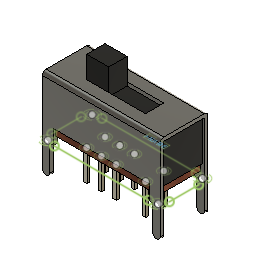
Switch-EG2301 v5 (Autodesk Fusion 360 design; units mm, degrees)
Autodesk Fusion 360 part; units mm, degrees
sketch "Sketch1" plane through (0, 0, 0) normal (0, 0, 1) x (1, 0, 0)
  line L0 (-4.25, 1.45) -> (-3.75, 1.45)
  line L1 (-3.75, 1.45) -> (-3.75, 1.05)
  line L2 (-3.75, 1.05) -> (-4.25, 1.05)
  line L3 (-4.25, 1.05) -> (-4.25, 1.45)
  line L4 (-2.25, 1.45) -> (-1.75, 1.45)
  line L5 (-1.75, 1.45) -> (-1.75, 1.05)
  line L6 (-1.75, 1.05) -> (-2.25, 1.05)
  line L7 (-2.25, 1.05) -> (-2.25, 1.45)
  line L8 (-0.25, 1.45) -> (0.25, 1.45)
  line L9 (0.25, 1.45) -> (0.25, 1.05)
  line L10 (0.25, 1.05) -> (-0.25, 1.05)
  line L11 (-0.25, 1.05) -> (-0.25, 1.45)
  line L12 (3.75, 1.45) -> (4.25, 1.45)
  line L13 (4.25, 1.45) -> (4.25, 1.05)
  line L14 (4.25, 1.05) -> (3.75, 1.05)
  line L15 (3.75, 1.05) -> (3.75, 1.45)
  line L16 (-8, 3.25) -> (-7, 3.25)
  line L17 (-7, 3.25) -> (-7, 2.75)
  line L18 (-7, 2.75) -> (-8, 2.75)
  line L19 (-8, 2.75) -> (-8, 3.25)
  line L20 (7, 3.25) -> (8, 3.25)
  line L21 (8, 3.25) -> (8, 2.75)
  line L22 (8, 2.75) -> (7, 2.75)
  line L23 (7, 2.75) -> (7, 3.25)
  line L24 (0, 0) -> (8, 0) construction
  line L25 (0.25, -1.45) -> (0.25, -1.05)
  line L26 (-2.25, -1.45) -> (-1.75, -1.45)
  line L27 (-0.25, -1.05) -> (-0.25, -1.45)
  line L28 (-8, -3.25) -> (-7, -3.25)
  line L29 (-3.75, -1.05) -> (-4.25, -1.05)
  line L30 (7, -3.25) -> (8, -3.25)
  line L31 (8, -2.75) -> (7, -2.75)
  line L32 (7, -2.75) -> (7, -3.25)
  line L33 (3.75, -1.05) -> (3.75, -1.45)
  line L34 (8, -3.25) -> (8, -2.75)
  line L35 (-0.25, -1.45) -> (0.25, -1.45)
  line L36 (-7, -2.75) -> (-8, -2.75)
  line L37 (-2.25, -1.05) -> (-2.25, -1.45)
  line L38 (-3.75, -1.45) -> (-3.75, -1.05)
  line L39 (-4.25, -1.45) -> (-3.75, -1.45)
  line L40 (-4.25, -1.05) -> (-4.25, -1.45)
  line L41 (0.25, -1.05) -> (-0.25, -1.05)
  line L42 (-7, -3.25) -> (-7, -2.75)
  line L43 (-1.75, -1.05) -> (-2.25, -1.05)
  line L44 (3.75, -1.45) -> (4.25, -1.45)
  line L45 (-8, -2.75) -> (-8, -3.25)
  line L46 (4.25, -1.05) -> (3.75, -1.05)
  line L47 (-1.75, -1.45) -> (-1.75, -1.05)
  line L48 (4.25, -1.45) -> (4.25, -1.05)
  dimension "d1" = 0.5
  dimension "d2" = 1
  dimension "d3" = 1
  dimension "d4" = 0.5
  dimension "d5" = 0.5
  dimension "d6" = 0.4
  dimension "d7" = 0.5
  dimension "d8" = 0.4
  dimension "d9" = 0.5
  dimension "d10" = 0.4
  dimension "d11" = 0.5
  dimension "d12" = 0.4
  dimension "d13" = 0.25
  dimension "d14" = 1.05
  dimension "d15" = 4.25
  dimension "d16" = 1.75
  dimension "d17" = 3.75
  dimension "d18" = 7
  dimension "d19" = 8
  dimension "d20" = 2.75
  constraint horizontal L0
  constraint vertical L1
  constraint horizontal L2
  constraint vertical L3
  constraint horizontal L4
  constraint vertical L5
  constraint horizontal L6
  constraint vertical L7
  constraint horizontal L8
  constraint vertical L9
  constraint horizontal L10
  constraint vertical L11
  constraint horizontal L12
  constraint vertical L13
  constraint horizontal L14
  constraint vertical L15
  constraint horizontal L16
  constraint vertical L17
  constraint horizontal L18
  constraint vertical L19
  constraint horizontal L20
  constraint vertical L21
  constraint horizontal L22
  constraint vertical L23
  constraint collinear L0 L4
  constraint collinear L4 L8
  constraint collinear L8 L12
  constraint collinear L16 L20
  constraint coincident L24.start origin
  constraint perpendicular L11 L24
  constraint symmetric L0.start L24 L39.start
  constraint symmetric L0.end L24 L38.start
  constraint symmetric L1.end L24 L29.start
  constraint symmetric L2.end L24 L29.end
  constraint symmetric L4.start L24 L26.start
  constraint symmetric L4.end L24 L26.end
  constraint symmetric L5.end L24 L43.start
  constraint symmetric L6.end L24 L37.start
  constraint symmetric L8.start L24 L27.end
  constraint symmetric L8.end L24 L25.start
  constraint symmetric L9.end L24 L25.end
  constraint symmetric L10.end L24 L27.start
  constraint symmetric L12.start L24 L33.end
  constraint symmetric L12.end L24 L44.end
  constraint symmetric L13.end L24 L46.start
  constraint symmetric L14.end L24 L33.start
  constraint symmetric L16.start L24 L28.start
  constraint symmetric L16.end L24 L28.end
  constraint symmetric L17.end L24 L36.start
  constraint symmetric L18.end L24 L36.end
  constraint symmetric L20.start L24 L30.start
  constraint symmetric L20.end L24 L30.end
  constraint symmetric L21.end L24 L31.start
  constraint symmetric L22.end L24 L31.end
  measures "d1" distance of L16.end L17.end
  measures "d2" distance of L16.start L16.end
  measures "d3" distance of L20.start L20.end
  measures "d4" distance of L20.end L21.end
  measures "d5" distance of L12.start L12.end
  measures "d6" distance of L12.end L13.end
  measures "d7" distance of L8.start L8.end
  measures "d8" distance of L8.end L9.end
  measures "d9" distance of L4.start L4.end
  measures "d10" distance of L4.end L5.end
  measures "d11" distance of L0.start L0.end
  measures "d12" distance of L0.end L1.end
  measures "d13" distance of L24.start L9
  measures "d14" distance of L24.start L10
  measures "d15" distance of L24.start L13
  measures "d16" distance of L24.start L5
  measures "d17" distance of L24.start L1
  measures "d18" distance of L24.start L17
  measures "d19" distance of L24.start L21
  measures "d20" distance of L24.start L22
extrude "Extrude1" add sketch "Sketch1" against normal blind 4 makes body 1 at (-0.0833, -1.45, -1.3333) makes body 2 at (7.6667, 2.75, -1.3333) makes body 3 at (-4.0833, 1.45, -1.3333) makes body 4 at (-2.0833, 1.45, -1.3333) makes body 5 at (-7.6667, -3.25, -1.3333) makes body 6 at (4.0833, -1.05, -1.3333) makes body 7 at (-2.0833, -1.45, -1.3333) makes body 8 at (4.0833, 1.05, -1.3333) makes body 9 at (-7.6667, 3.25, -1.3333) makes body 10 at (-0.0833, 1.45, -1.3333) makes body 11 at (-4.0833, -1.45, -1.3333) makes body 12 at (7.6667, -2.75, -1.3333)
fillet "Fillet1" radius 0.5 8 edges at (8, 3, -4) (7, 3, -4) (-7, -3, -4) (-8, -3, -4) (-7, 3, -4) (-8, 3, -4) (8, -3, -4) (7, -3, -4) on bodies 2 5 9 12
sketch "Sketch2" plane through (0, 0, 0) normal (0, 0, 1) x (1, 0, 0)
  line L0 (-8, 2.75) -> (-7, 2.75)
  line L1 (-7, 2.75) -> (-7, 3.25)
  line L2 (-7, 3.25) -> (-8, 3.25)
  line L3 (-8, 3.25) -> (-8, 2.75)
  line L4 (-4.25, 1.05) -> (-3.75, 1.05)
  line L5 (-3.75, 1.05) -> (-3.75, 1.45)
  line L6 (-3.75, 1.45) -> (-4.25, 1.45)
  line L7 (-4.25, 1.45) -> (-4.25, 1.05)
  line L8 (-2.25, 1.05) -> (-1.75, 1.05)
  line L9 (-1.75, 1.05) -> (-1.75, 1.45)
  line L10 (-1.75, 1.45) -> (-2.25, 1.45)
  line L11 (-2.25, 1.45) -> (-2.25, 1.05)
  line L12 (-0.25, 1.05) -> (0.25, 1.05)
  line L13 (0.25, 1.05) -> (0.25, 1.45)
  line L14 (0.25, 1.45) -> (-0.25, 1.45)
  line L15 (-0.25, 1.45) -> (-0.25, 1.05)
  line L16 (0.25, -1.05) -> (-0.25, -1.05)
  line L17 (-0.25, -1.05) -> (-0.25, -1.45)
  line L18 (-0.25, -1.45) -> (0.25, -1.45)
  line L19 (0.25, -1.45) -> (0.25, -1.05)
  line L20 (-1.75, -1.45) -> (-1.75, -1.05)
  line L21 (-1.75, -1.05) -> (-2.25, -1.05)
  line L22 (-2.25, -1.05) -> (-2.25, -1.45)
  line L23 (-2.25, -1.45) -> (-1.75, -1.45)
  line L24 (-4.25, -1.05) -> (-4.25, -1.45)
  line L25 (-4.25, -1.45) -> (-3.75, -1.45)
  line L26 (-3.75, -1.45) -> (-3.75, -1.05)
  line L27 (-3.75, -1.05) -> (-4.25, -1.05)
  line L28 (3.75, 1.05) -> (4.25, 1.05)
  line L29 (4.25, 1.05) -> (4.25, 1.45)
  line L30 (4.25, 1.45) -> (3.75, 1.45)
  line L31 (3.75, 1.45) -> (3.75, 1.05)
  line L32 (7, 2.75) -> (8, 2.75)
  line L33 (8, 2.75) -> (8, 3.25)
  line L34 (8, 3.25) -> (7, 3.25)
  line L35 (7, 3.25) -> (7, 2.75)
  line L36 (4.25, -1.45) -> (4.25, -1.05)
  line L37 (4.25, -1.05) -> (3.75, -1.05)
  line L38 (3.75, -1.05) -> (3.75, -1.45)
  line L39 (3.75, -1.45) -> (4.25, -1.45)
  line L40 (8, -3.25) -> (8, -2.75)
  line L41 (8, -2.75) -> (7, -2.75)
  line L42 (7, -2.75) -> (7, -3.25)
  line L43 (7, -3.25) -> (8, -3.25)
  line L44 (-8, -2.75) -> (-8, -3.25)
  line L45 (-8, -3.25) -> (-7, -3.25)
  line L46 (-7, -3.25) -> (-7, -2.75)
  line L47 (-7, -2.75) -> (-8, -2.75)
  line L48 (7, 3.25) -> (6.5, 3.25)
  line L49 (6.5, 3.25) -> (6.5, 2.75)
  line L50 (6.5, 2.75) -> (7, 2.75)
  line L51 (7, 2.75) -> (7, 3.25)
  line L52 (0, 0) -> (0.107, 0) construction
  line L53 (0.107, 0) -> (7.5, 0) construction
  line L54 (0, 0) -> (0, 3) construction
  line L55 (-6.5, 2.75) -> (-7, 2.75)
  line L56 (-6.5, 3.25) -> (-6.5, 2.75)
  line L57 (-7, 3.25) -> (-6.5, 3.25)
  line L58 (-7, 2.75) -> (-7, 3.25)
  line L59 (-6.5, -2.75) -> (-7, -2.75)
  line L60 (-7, -3.25) -> (-6.5, -3.25)
  line L61 (-7, -2.75) -> (-7, -3.25)
  line L62 (-7, -2.75) -> (-7, -3.25)
  line L63 (-6.5, -3.25) -> (-6.5, -2.75)
  line L64 (6.5, -3.25) -> (6.5, -2.75)
  line L65 (7, -2.75) -> (7, -3.25)
  line L66 (7, -3.25) -> (7, -2.75)
  line L67 (6.5, -2.75) -> (7, -2.75)
  line L68 (7, -3.25) -> (6.5, -3.25)
  dimension "d25" = 0.5
  constraint horizontal L48
  constraint vertical L49
  constraint horizontal L50
  constraint vertical L51
  constraint coincident L34.end L35.start
  constraint collinear L32 L50
  constraint coincident L52.start L54.start
  constraint perpendicular L38 L52
  constraint perpendicular L38 L53
  constraint perpendicular L52 L54
  constraint symmetric L34.end L54 L1.end
  constraint symmetric L48.end L54 L56.start
  constraint symmetric L49.end L54 L55.start
  constraint symmetric L32.start L54 L0.end
  constraint symmetric L0.end L53 L46.end
  constraint symmetric L1.end L53 L45.end
  constraint symmetric L32.start L53 L41.end
  constraint symmetric L34.end L53 L42.end
  constraint symmetric L48.end L53 L64.start
  constraint symmetric L49.end L53 L64.end
  constraint symmetric L53 L55.start L59.start
  constraint symmetric L53 L0.end L46.end
  constraint symmetric L53 L56.start L60.end
  constraint symmetric L53 L1.end L45.end
  measures "d25" distance of L34.end L48.end
extrude "Extrude2" add sketch "Sketch2" along normal blind 1 bodies 1 2 3 4 5 6 7 8 9 10 11 12
sketch "Sketch3" plane through (0, 0, 1) normal (0, 0, 1) x (-1, 0, 0)
  line L0 (-0.25, 1.45) -> (-0.25, 1.05)
  line L1 (-0.25, 1.05) -> (0.25, 1.05)
  line L2 (0.25, 1.05) -> (0.25, 1.45)
  line L3 (0.25, 1.45) -> (-0.25, 1.45)
  line L4 (7.5, -3) -> (-7.5, -3)
  line L5 (-7.5, -3) -> (-7.5, 3)
  line L6 (-7.5, 3) -> (7.5, 3)
  line L7 (7.5, 3) -> (7.5, -3)
  line L8 (8, -3.25) -> (8, -2.75)
  line L9 (8, -2.75) -> (6.5, -2.75)
  line L10 (6.5, -2.75) -> (6.5, -3.25)
  line L11 (6.5, -3.25) -> (8, -3.25)
  line L12 (-6.5, -2.75) -> (-8, -2.75)
  line L13 (-8, -2.75) -> (-8, -3.25)
  line L14 (-8, -3.25) -> (-6.5, -3.25)
  line L15 (-6.5, -3.25) -> (-6.5, -2.75)
  line L16 (-8, 3.25) -> (-8, 2.75)
  line L17 (-8, 2.75) -> (-6.5, 2.75)
  line L18 (-6.5, 2.75) -> (-6.5, 3.25)
  line L19 (-6.5, 3.25) -> (-8, 3.25)
  line L20 (6.5, 3.25) -> (6.5, 2.75)
  line L21 (6.5, 2.75) -> (8, 2.75)
  line L22 (8, 2.75) -> (8, 3.25)
  line L23 (8, 3.25) -> (6.5, 3.25)
  dimension "d28" = 7.5
  dimension "d29" = 7.5
  dimension "d30" = 3
  dimension "d31" = 3
  constraint horizontal L4
  constraint vertical L5
  constraint horizontal L6
  constraint vertical L7
  measures "d28" distance of origin L5
  measures "d29" distance of origin L7
  measures "d30" distance of origin L4
  measures "d31" distance of origin L6
extrude "Extrude3" add sketch "Sketch3" along normal blind 1 contours L0 L1 L2 L3 | L4 L7 L8 L9 L10 L11 | L4 L7 L9 L10 | L4 L5 L6 L7 L9 L10 L12 L15 L17 L18 L20 L21 | L4 L5 L12 L13 L14 L15 | L4 L5 L12 L15 | L6 L7 L20 L21 | L6 L7 L20 L21 L22 L23 | L5 L6 L16 L17 L18 L19 | L5 L6 L17 L18 bodies 1 2 3 4 5 6 7 8 9 10 11 12
sketch "Sketch4" plane through (0, 0, 2) normal (0, 0, 1) x (-1, 0, 0)
  line L0 (7.5, 2.75) -> (8, 2.75)
  line L1 (8, 2.75) -> (8, 3.25)
  line L2 (8, 3.25) -> (6.5, 3.25)
  line L3 (6.5, 3.25) -> (6.5, 3)
  line L4 (6.5, 3) -> (-6.5, 3)
  line L5 (-6.5, 3) -> (-6.5, 3.25)
  line L6 (-6.5, 3.25) -> (-8, 3.25)
  line L7 (-8, 3.25) -> (-8, 2.75)
  line L8 (-8, 2.75) -> (-7.5, 2.75)
  line L9 (-7.5, 2.75) -> (-7.5, -2.75)
  line L10 (-7.5, -2.75) -> (-8, -2.75)
  line L11 (-8, -2.75) -> (-8, -3.25)
  line L12 (-8, -3.25) -> (-6.5, -3.25)
  line L13 (-6.5, -3.25) -> (-6.5, -3)
  line L14 (-6.5, -3) -> (6.5, -3)
  line L15 (6.5, -3) -> (6.5, -3.25)
  line L16 (6.5, -3.25) -> (8, -3.25)
  line L17 (8, -3.25) -> (8, -2.75)
  line L18 (8, -2.75) -> (7.5, -2.75)
  line L19 (7.5, -2.75) -> (7.5, 2.75)
  line L20 (6.5, -3.25) -> (-6.5, -3.25)
  line L21 (-7.75, -2.75) -> (-7.75, 2.75)
  line L22 (-6.5, 3.25) -> (6.5, 3.25)
  line L23 (7.75, 2.75) -> (7.75, -2.75)
  constraint coincident L15.end L16.start
  constraint coincident L12.end L13.start
  constraint midpoint L10 L21.start
  constraint midpoint L8 L21.end
  constraint coincident L5.end L6.start
  constraint coincident L2.end L3.start
  constraint midpoint L0 L23.start
  constraint midpoint L18 L23.end
extrude "Extrude4" add sketch "Sketch4" along normal blind 5.5 bodies 1
sketch "Sketch5" plane through (0, 0, 7.5) normal (0, 0, 1) x (-1, 0, 0)
  line L0 (8, 2.75) -> (8, 3.25)
  line L1 (8, 3.25) -> (-8, 3.25)
  line L2 (-8, 3.25) -> (-8, 2.75)
  line L3 (-8, 2.75) -> (-7.75, 2.75)
  line L4 (-7.75, 2.75) -> (-7.75, -2.75)
  line L5 (-7.75, -2.75) -> (-8, -2.75)
  line L6 (-8, -2.75) -> (-8, -3.25)
  line L7 (-8, -3.25) -> (8, -3.25)
  line L8 (8, -3.25) -> (8, -2.75)
  line L9 (8, -2.75) -> (7.75, -2.75)
  line L10 (7.75, -2.75) -> (7.75, 2.75)
  line L11 (7.75, 2.75) -> (8, 2.75)
  line L12 (8, -3.25) -> (-8, -3.25)
  line L13 (-8, -3.25) -> (-8, 3.25)
  line L14 (-8, 3.25) -> (8, 3.25)
  line L15 (8, 3.25) -> (8, -3.25)
  line L16 (4, -1.25) -> (-4, -1.25)
  line L17 (-4, -1.25) -> (-4, 1.25)
  line L18 (-4, 1.25) -> (4, 1.25)
  line L19 (4, 1.25) -> (4, -1.25)
  line L20 (1, -1.25) -> (1, 1.25)
  dimension "d36" = 8
  dimension "d37" = 2.5
  dimension "d38" = 1.25
  dimension "d39" = 4
  dimension "d40" = 3
  constraint horizontal L12
  constraint vertical L13
  constraint horizontal L14
  constraint vertical L15
  constraint coincident L1.end L2.start
  constraint coincident L7.end L8.start
  constraint horizontal L16
  constraint vertical L17
  constraint horizontal L18
  constraint vertical L19
  constraint coincident L16 L20.start
  constraint coincident L18 L20.end
  constraint perpendicular L18 L20
  measures "d36" distance of L16.start L16.end
  measures "d37" distance of L16.end L17.end
  measures "d38" distance of origin L16
  measures "d39" distance of origin L19
  measures "d40" distance of L19 L20
extrude "Extrude5" add sketch "Sketch5" along normal blind 0.5 contours L0 L1 L2 L3 L4 L5 L6 L7 L8 L9 L10 L11 L12 L13 L14 L15 | L16 L18 L19 L20 bodies 1
sketch "Sketch6" plane through (0, 0, 8) normal (0, 0, 1) x (-1, 0, 0)
  line L0 (1, -1.25) -> (-4, -1.25)
  line L1 (-4, -1.25) -> (-4, 1.25)
  line L2 (-4, 1.25) -> (1, 1.25)
  line L3 (1, 1.25) -> (1, -1.25)
  line L4 (-8, 2.75) -> (-7.75, 2.75)
  line L5 (-7.75, 2.75) -> (-7.75, -2.75)
  line L6 (-7.75, -2.75) -> (-8, -2.75)
  line L7 (-8, -2.75) -> (-8, -3.25)
  line L8 (-8, -3.25) -> (8, -3.25)
  line L9 (8, -3.25) -> (8, -2.75)
  line L10 (8, -2.75) -> (7.75, -2.75)
  line L11 (7.75, -2.75) -> (7.75, 2.75)
  line L12 (7.75, 2.75) -> (8, 2.75)
  line L13 (8, 2.75) -> (8, 3.25)
  line L14 (8, 3.25) -> (-8, 3.25)
  line L15 (-8, 3.25) -> (-8, 2.75)
  line L16 (1, -1.25) -> (4, -1.25)
  line L17 (4, -1.25) -> (4, 1.25)
  line L18 (4, 1.25) -> (1, 1.25)
  line L19 (1, 1.25) -> (1, -1.25)
  dimension "d43" = 3
  constraint horizontal L16
  constraint vertical L17
  constraint horizontal L18
  constraint vertical L19
  constraint coincident L0.start L3.end
  constraint collinear L2 L18
  measures "d43" distance of L0.start L16.end
extrude "Extrude6" add sketch "Sketch6" along normal blind 3 contours L3 L16 L17 L18 L19 bodies 1
sketch "Sketch7" plane through (0, 0, 7.5) normal (0, 0, 1) x (-1, 0, 0)
  line L0 (4, -1.25) -> (1, -1.25)
  line L1 (1, -1.25) -> (-4, -1.25)
  line L2 (-4, -1.25) -> (-4, 1.25)
  line L3 (-4, 1.25) -> (1, 1.25)
  line L4 (1, 1.25) -> (4, 1.25)
  line L5 (4, 1.25) -> (4, -1.25)
  line L6 (-8, 2.75) -> (-7.75, 2.75)
  line L7 (-7.75, 2.75) -> (-7.75, -2.75)
  line L8 (-7.75, -2.75) -> (-8, -2.75)
  line L9 (-8, -2.75) -> (-8, -3.25)
  line L10 (-8, -3.25) -> (8, -3.25)
  line L11 (8, -3.25) -> (8, -2.75)
  line L12 (8, -2.75) -> (7.75, -2.75)
  line L13 (7.75, -2.75) -> (7.75, 2.75)
  line L14 (7.75, 2.75) -> (8, 2.75)
  line L15 (8, 2.75) -> (8, 3.25)
  line L16 (8, 3.25) -> (-8, 3.25)
  line L17 (-8, 3.25) -> (-8, 2.75)
  line L18 (8, -2.75) -> (8, 2.75)
  line L19 (-8, -2.75) -> (-8, 2.75)
  constraint coincident L11.end L12.start
  constraint coincident L14.end L15.start
  constraint coincident L8.end L9.start
  constraint coincident L6.start L17.end
extrude "Extrude8" add sketch "Sketch7" along normal blind 0.5 contours L6 L7 L8 L19 | L12 L13 L14 L18 bodies 1
fillet "Fillet2" radius 0.5 2 edges at (0, -3.25, 8) (0, 3.25, 8) on bodies 1
extrude "Extrude7" [suppressed]
